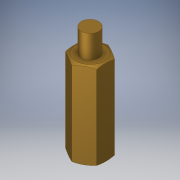
# Autodesk Inventor part: espaçador 15mm m3
Saved by Autodesk Inventor 2019.4 (Build 234330000, 330)
## iProperties
Created: 2021-02-09
Part Number: espaçador 15mm m3
Material: Aço galvanizado
Document SubType Name: Modeling
Designer: Lattes
Density: 7.85 g/cm^3
Appearance: Latão - Acetinado
Author: Lattes
Autodesk Inventor part; units mm, degrees
ref_plane "YZ Plane" through (0, 0, 0) normal (1, 0, 0) x (0, 1, 0)
ref_plane "XZ Plane" through (0, 0, 0) normal (0, 1, 0) x (-1, 0, 0)
ref_plane "XY Plane" through (0, 0, 0) normal (0, 0, 1) x (1, 0, 0)
sketch "Esboço2" plane through (0, 0, 0) normal (0, 1, 0) x (-1, 0, 0)
  circle A0 centre (0, 0) radius 1.5
  line L0 (2.7, -1.5588) -> (0, -3.1177)
  line L1 (0, -3.1177) -> (-2.7, -1.5588)
  line L2 (-2.7, -1.5588) -> (-2.7, 1.5588)
  line L3 (-2.7, 1.5588) -> (0, 3.1177)
  line L4 (0, 3.1177) -> (2.7, 1.5588)
  line L5 (2.7, 1.5588) -> (2.7, -1.5588)
  constraints: 12 end point, 1 centre point
extrude "Extrusão1" add sketch "Esboço2" along normal blind 15
thread "Rosca1" size "M3x0.5" class "6H" standard "ANSI Metric M Profile" full length
chamfer "Chanfro1" distance 0.3 angle 45 2 edges at (1.5, 15, 0) (1.5, 0, 0)
sketch "Esboço3" plane through (0, 0, 0) normal (0, 0, 1) x (1, 0, 0)
  line L0 (0, -0.48) -> (0, 2.88) projected
  line L1 (2.4, 0) -> (4.5158, 0.9866)
  line L2 (2.4, 0) -> (4.5158, 0.9866)
  line L3 (4.5158, 0.9866) -> (4.5158, 0)
  line L4 (4.5158, 0.9866) -> (2.4, 0)
  line L5 (2.4, 0) -> (4.5158, 0)
  line L6 (2.7, 0) -> (0, 0) projected
  line L7 (2.4, 2.4) -> (2.4, 15.0122)
  line L8 (4.5158, 15.0122) -> (2.4, 15.0122)
  line L9 (4.5158, 15.0122) -> (4.5158, 14.0252)
  line L10 (4.5158, 14.0252) -> (2.4, 15.0122)
  dimension "d19" = 0.987
  constraints: 18 end point, 2 collinear, 1 vertical
  measures "d19" distance of L8.start L9.end
revolve "Revolução3" cut sketch "Esboço3" angle 360 about axis through (0, -10, 0) along (0, 1, 0)
sketch "Esboço4" plane through (0, 15, 0) normal (0, 1, 0) x (1, 0, 0)
  circle A0 centre (0, 0) radius 2.4262
  constraints: 1 centre point, 1 coincident
extrude "Extrusão2" add sketch "Esboço4" against normal blind 1.5
sketch "Esboço5" plane through (0, 15, 0) normal (0, 1, 0) x (1, 0, 0)
  circle A0 centre (0, 0) radius 1.5
  dimension "d23" = 3
  constraints: 1 centre point, 1 coincident
  measures "d23" diameter of A0
extrude "Extrusão3" add sketch "Esboço5" along normal blind 4
